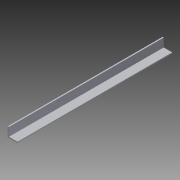
# Autodesk Inventor part: Bumper Metal Edge Part3 (24x28 robot)
Saved by Autodesk Inventor 2013 (Build 170138000, 138)
## iProperties
Created: 2013-01-06
Part Number: Bumper Metal Edge Part3 (24x28 robot)
Material: Aluminum 6061
Document SubType Name: Modeling
Designer: Moses
Mass: 20.6541 g
Surface Area: 103.175 cm^2
Volume: 7.62143 cm^3
Density: 2.71 g/cm^3
Author: Moses
Autodesk Inventor part; units mm, degrees
ref_plane "YZ Plane" through (0, 0, 0) normal (1, 0, 0) x (0, 1, 0)
ref_plane "XZ Plane" through (0, 0, 0) normal (0, 1, 0) x (-1, 0, 0)
ref_plane "XY Plane" through (0, 0, 0) normal (0, 0, 1) x (1, 0, 0)
sketch "Sketch1" plane through (0, 0, 0) normal (0, 0, 1) x (1, 0, 0)
  line L0 (0, 0) -> (0, 12.7)
  line L1 (0, 12.7) -> (1.5875, 12.7)
  line L2 (0, 0) -> (12.7, 0)
  line L3 (12.7, 0) -> (12.7, 1.5875)
  line L4 (12.7, 1.5875) -> (1.5875, 1.5875)
  line L5 (1.5875, 1.5875) -> (1.5875, 12.7)
  dimension "d0" = 12.7
  dimension "d1" = 1.5875
  dimension "d2" = 12.7
  dimension "d3" = 1.5875
  constraints: 12 end point, 3 parallel, 2 perpendicular, 1 vertical
  measures "d0" distance of L0.start L0.end
  measures "d1" distance of L0.end L1.end
  measures "d2" distance of L0.start L2.end
  measures "d3" distance of L2.end L3.end
extrude "Extrusion1" add sketch "Sketch1" along normal blind 201.6125
body "Solid1"
